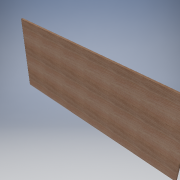
# Autodesk Inventor part: tablero_granded
Saved by Autodesk Inventor 2016 (Build 200138000, 138)
## iProperties
Created: 2018-06-24
Part Number: tablero_granded
Material: Wood (Birch)
Document SubType Name: Modeling
Designer: damia
Density: 0.55 g/cm^3
Appearance: Birch - Natural Polished
Mass: 10195.8 g
Surface Area: 21401.5 cm^2
Volume: 18537.9 cm^3
Author: damia
Autodesk Inventor part; units mm, degrees
ref_plane "YZ Plane" through (0, 0, 0) normal (1, 0, 0) x (0, 1, 0)
ref_plane "XZ Plane" through (0, 0, 0) normal (0, 1, 0) x (-1, 0, 0)
ref_plane "XY Plane" through (0, 0, 0) normal (0, 0, 1) x (1, 0, 0)
sketch "Sketch2" plane through (0, 0, 0) normal (0, 1, 0) x (-1, 0, 0)
  line L0 (0, 0) -> (-1582, 0)
  line L1 (-1582, 0) -> (-1582, -651)
  line L2 (-1582, -651) -> (0, -651)
  line L3 (0, -651) -> (0, 0)
  dimension "d4" = 1582
  dimension "d5" = 651
  constraints: 8 end point, 2 parallel, 1 horizontal, 1 perpendicular
  measures "d4" distance of L2.end L1.end
  measures "d5" distance of L1.end L0.end
extrude "Extrusion2" add sketch "Sketch2" along normal blind 18
equation "\"d5\" = Profundidad"
equation "\"Profundidad\" = 651"
body "Solid2"
